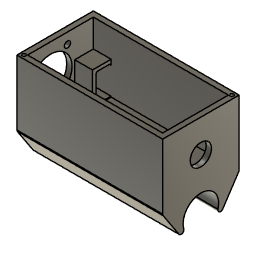
controller box (Autodesk Fusion 360 design; units mm, degrees)
Autodesk Fusion 360 part; units mm, degrees
note: some values were not read from the file. Set by a fixed rule: which sketch regions a step uses.
sketch "Sketch1" plane through (0, 0, 0) normal (0, 0, 1) x (1, 0, 0)
  line L0 (0, 0) -> (82, 0)
  line L1 (82, 0) -> (82, 43)
  line L2 (82, 43) -> (0, 43)
  line L3 (0, 43) -> (0, 0)
  dimension "d1" = 82
  dimension "d2" = 43
  constraint horizontal L0
  constraint vertical L1
  constraint horizontal L2
  constraint vertical L3
  constraint coincident L0.start L3.end
  measures "d1" distance of L0.start L0.end
  measures "d2" distance of L0.start L2.end
extrude "Extrude1" add sketch "Sketch1" along normal blind 37
sketch "Sketch2" plane through (0, 0, 37) normal (0, 0, 1) x (-1, 0, 0)
  line L0 (0, -43) -> (0, 0)
  line L1 (0, 0) -> (-82, 0)
  line L2 (-82, 0) -> (-82, -43)
  line L3 (-82, -43) -> (0, -43)
  line L4 (-3, -3) -> (-79, -3)
  line L5 (-79, -3) -> (-79, -40)
  line L6 (-79, -40) -> (-3, -40)
  line L7 (-3, -40) -> (-3, -3)
  dimension "d5" = 3
  dimension "d6" = 3
  dimension "d7" = 3
  dimension "d8" = 3
  constraint horizontal L4
  constraint vertical L5
  constraint horizontal L6
  constraint vertical L7
  measures "d5" distance of L3 L6
  measures "d6" distance of L0 L7
  measures "d7" distance of L1 L4
  measures "d8" distance of L2 L5
extrude "Extrude2" cut sketch "Sketch2" against normal blind 34 contours L4 L5 L6 L7
sketch "Sketch3" plane through (0, 0, 0) normal (-1, 0, 0) x (0, -1, 0)
  line L0 (-43, 0) -> (0, 0)
  line L1 (0, 0) -> (0, 37)
  line L2 (0, 37) -> (-43, 37)
  line L3 (-43, 37) -> (-43, 0)
  circle A0 centre (-21.5, -10) radius 10
  circle A1 centre (-21.5, -10) radius 12.5
  line L4 (-46.7088, -16) -> (3.2912, -16)
  line L5 (-32.4659, -16) -> (-43, 0)
  line L6 (-10.5341, -16) -> (0, 0)
  dimension "d11" = 20
  dimension "d12" = 25
  dimension "d13" = 10
  dimension "d14" = 21.5
  dimension "d16" = 16
  constraint concentric A0 A1
  constraint horizontal L4
  constraint coincident A1 L5.start
  constraint coincident L4 L5.start
  constraint coincident L0.start L3.end
  constraint coincident A1 L6.start
  constraint coincident L4 L6.start
  constraint coincident L0.end L1.start
  measures "d11" diameter of A0
  measures "d12" diameter of A1
  measures "d13" distance of L0 A0.centre
  measures "d14" distance of L1 A0.centre
  measures "d16" distance of L0 L4
extrude "Extrude3" add sketch "Sketch3" against normal blind 82 contours L0 A1 L5 | L0 A0 A1 L4 | L0 A0 A1 L4 | L0 A1 L6
fillet "Fillet1" radius 1.5 6 edges at (41, 13.5, -16) (41, 29.5, -16) (41, 32.4659, -16) (41, 10.5341, -16) (41, 43, 0) (41, 0, 0)
sketch "Sketch4" plane through (0, 0, 0) normal (-1, 0, 0) x (0, -1, 0)
  arc A0 (-0.2472, -0.3754) -> (0, 0.4495) centre (-1.5, 0.4495) ccw
  line L0 (0, 0.4495) -> (0, 37)
  line L1 (0, 37) -> (-43, 37)
  line L2 (-43, 37) -> (-43, 0.4495)
  arc A1 (-43, 0.4495) -> (-42.7528, -0.3754) centre (-41.5, 0.4495) ccw
  line L3 (-42.7528, -0.3754) -> (-33.8235, -13.938)
  arc A2 (-33.8235, -13.938) -> (-31.1266, -12.7071) centre (-32.5706, -13.1131) ccw
  arc A3 (-11.8734, -12.7071) -> (-31.1266, -12.7071) centre (-21.5, -10) ccw
  arc A4 (-11.8734, -12.7071) -> (-9.1765, -13.938) centre (-10.4294, -13.1131) ccw
  line L4 (-9.1765, -13.938) -> (-0.2472, -0.3754)
  line L5 (-29, 34.4495) -> (-3, 34.4495)
  line L6 (-3, 34.4495) -> (-3, 3.4495)
  line L7 (-3, 3.4495) -> (-29, 3.4495)
  line L8 (-29, 3.4495) -> (-29, 34.4495)
  circle A5 centre (-16, 18.9495) radius 12
  circle A6 centre (-25.45, 30.8995) radius 1.75
  circle A7 centre (-6.55, 6.9995) radius 1.75
  line L9 (0, 0.4495) -> (-43, 0.4495)
  line L10 (-31.5, 3.4495) -> (-40, 3.4495)
  line L11 (-40, 3.4495) -> (-40, 19.4495)
  line L12 (-40, 19.4495) -> (-31.5, 19.4495)
  line L13 (-31.5, 19.4495) -> (-31.5, 3.4495)
  dimension "d21" = 24
  dimension "d22" = 31
  dimension "d23" = 26
  dimension "d24" = 13
  dimension "d25" = 15.5
  dimension "d26" = 3.5
  dimension "d27" = 3.5
  dimension "d28" = 3.55
  dimension "d29" = 3.55
  dimension "d30" = 3.55
  dimension "d31" = 3.55
  dimension "d32" = 3
  dimension "d33" = 3
  dimension "d34" = 16
  dimension "d35" = 8.5
  dimension "d36" = 3
  dimension "d37" = 3
  constraint horizontal L5
  constraint vertical L6
  constraint horizontal L7
  constraint vertical L8
  constraint coincident A0.end L0.start
  constraint coincident L2.end A1.start
  constraint horizontal L10
  constraint vertical L11
  constraint horizontal L12
  constraint vertical L13
  measures "d21" diameter of A5
  measures "d22" distance of L5.end L6.end
  measures "d23" distance of L5.start L5.end
  measures "d24" distance of L6 A5.centre
  measures "d25" distance of L5 A5.centre
  measures "d26" diameter of A6
  measures "d27" diameter of A7
  measures "d28" distance of L6 A7.centre
  measures "d29" distance of L7 A7.centre
  measures "d30" distance of L5 A6.centre
  measures "d31" distance of L8 A6.centre
  measures "d32" distance of L0 L6
  measures "d33" distance of L7 L9
  measures "d34" distance of L10.end L11.end
  measures "d35" distance of L11.end L12.end
  measures "d36" distance of L2 L11
  measures "d37" distance of L9 L10
extrude "Extrude4" cut sketch "Sketch4" against normal blind 3 contours A5 | A6 | A7 | L10 L11 L12 L13
sketch "Sketch5" plane through (3, 0, 0) normal (1, 0, 0) x (0, 1, 0)
  line L0 (40, 3.4495) -> (31.5, 3.4495)
  line L1 (31.5, 3.4495) -> (31.5, 19.4495)
  line L2 (31.5, 19.4495) -> (40, 19.4495)
  line L3 (40, 19.4495) -> (40, 37)
  line L4 (40, 37) -> (3, 37)
  line L5 (3, 37) -> (3, 3)
  line L6 (3, 3) -> (40, 3)
  line L7 (40, 3) -> (40, 3.4495)
  circle A0 centre (16, 18.9495) radius 12
  circle A1 centre (6.55, 6.9995) radius 1.75
  circle A2 centre (25.45, 30.8995) radius 1.75
  line L8 (40, 3) -> (29.5, 3)
  line L9 (29.5, 3) -> (29.5, 21.4495)
  line L10 (29.5, 21.4495) -> (40, 21.4495)
  line L11 (40, 21.4495) -> (40, 3)
  dimension "d40" = 2
  dimension "d41" = 2
  constraint horizontal L8
  constraint vertical L9
  constraint horizontal L10
  constraint vertical L11
  constraint coincident L6.end L7.start
  measures "d40" distance of L2 L10
  measures "d41" distance of L1 L9
extrude "Extrude5" add sketch "Sketch5" along normal blind 10 contours L0 L1 L2 L3 L6 L7 L8 L9 L10 L11
fillet "Fillet2" radius 1 2 edges at (6.5, 31.5, 19.4495) (6.5, 40, 19.4495)
sketch "Sketch6" plane through (82, 0, 0) normal (1, 0, 0) x (0, 1, 0)
  arc A0 (0, 0.4495) -> (0.2472, -0.3754) centre (1.5, 0.4495) ccw
  line L0 (0.2472, -0.3754) -> (9.1765, -13.938)
  arc A1 (9.1765, -13.938) -> (11.8734, -12.7071) centre (10.4294, -13.1131) ccw
  arc A2 (31.1266, -12.7071) -> (11.8734, -12.7071) centre (21.5, -10) ccw
  arc A3 (31.1266, -12.7071) -> (33.8235, -13.938) centre (32.5706, -13.1131) ccw
  line L1 (33.8235, -13.938) -> (42.7528, -0.3754)
  arc A4 (42.7528, -0.3754) -> (43, 0.4495) centre (41.5, 0.4495) ccw
  line L2 (43, 0.4495) -> (43, 37)
  line L3 (43, 37) -> (0, 37)
  line L4 (0, 37) -> (0, 0.4495)
  circle A5 centre (21.5, 18.725) radius 6
  dimension "d46" = 21.5
  dimension "d47" = 36.5505
  dimension "d48" = 18.275
  dimension "d49" = 12
  measures "d46" distance of L2 A5.centre
  measures "d47" distance of A4.end L2.end
  measures "d48" distance of L3 A5.centre
  measures "d49" diameter of A5
extrude "Extrude6" cut sketch "Sketch6" against normal blind 3 contours A5
sketch "Sketch7" plane through (0, 0, 37) normal (0, 0, 1) x (-1, 0, 0)
  line L0 (-79, -3) -> (-3, -3)
  line L1 (-3, -3) -> (-3, -40)
  line L2 (-3, -40) -> (-79, -40)
  line L3 (-79, -40) -> (-79, -3)
  line L4 (0, -43) -> (0, 0)
  line L5 (0, 0) -> (-82, 0)
  line L6 (-82, 0) -> (-82, -43)
  line L7 (-82, -43) -> (0, -43)
  circle A0 centre (-2, -2) radius 1
  circle A1 centre (-80, -41) radius 1
  dimension "d52" = 2
  dimension "d53" = 2
  dimension "d54" = 2
  dimension "d55" = 2
  dimension "d56" = 2
  dimension "d57" = 2
  measures "d52" diameter of A0
  measures "d53" distance of L5 A0.centre
  measures "d54" distance of L4 A0.centre
  measures "d55" diameter of A1
  measures "d56" distance of L6 A1.centre
  measures "d57" distance of L7 A1.centre
extrude "Extrude7" cut sketch "Sketch7" against normal blind 5 contours A0 | A1
equation "d14 = ( 43 / 2 ) * 1 mm"
equation "d24 = ( 26 / 2 ) * 1 mm"
equation "d25 = ( 31 / 2 ) * 1 mm"
equation "d46 = ( 43 / 2 ) * 1 mm"
equation "d48 = ( 36.55 / 2 ) * 1 mm"
